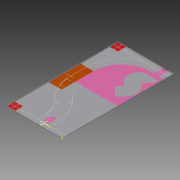
# Autodesk Inventor part: フィールド
Saved by Autodesk Inventor 2015 (Build 190159000, 159)
## iProperties
Created: 2015-08-24
Part Number: フィールド
Material: 一般
Document SubType Name: Modeling
Designer: nobuhiro
Density: 1 g/cm^3
Appearance: 既定
Author: nobuhiro
Autodesk Inventor part; units mm, degrees
ref_plane "YZ Plane" through (0, 0, 0) normal (1, 0, 0) x (0, 1, 0)
ref_plane "XZ Plane" through (0, 0, 0) normal (0, 1, 0) x (-1, 0, 0)
ref_plane "XY Plane" through (0, 0, 0) normal (0, 0, 1) x (1, 0, 0)
sketch "スケッチ1" plane through (0, 0, 0) normal (0, 0, 1) x (1, 0, 0)
  line L0 (7055, 13900) -> (-6950, 13900)
  line L1 (-6950, 13900) -> (-6950, 0)
  line L2 (-7000, -50) -> (0, -50)
  line L3 (0, 13950) -> (-7000, 13950)
  line L4 (-7000, 13950) -> (-7000, -50)
  line L5 (-25, 0) -> (0, 0)
  line L6 (130, 13900) -> (-25, 13900)
  line L7 (-25, 13900) -> (-25, 0)
  line L8 (0, -50) -> (0, 13950)
  line L9 (-6950, 0) -> (0, 0)
  point P0 (52.5, 13900)
  point P1 (52.5, 13900)
  dimension "d4" = 50
  dimension "d17" = 50
  dimension "d18" = 25
  dimension "d176" = 50
  dimension "d177" = 14000
  dimension "d178" = 7000
  constraints: 20 end point, 3 coincident, 3 parallel, 3 point on line, 2 horizontal, 2 midpoint
  measures "d4" distance between parallel lines of L3 L0
  measures "d17" distance between parallel lines of L2 L9
  measures "d18" distance between parallel lines of L8 L7
  measures "d176" distance between parallel lines of L4 L1
  measures "d177" distance of L3.end L2.start
  measures "d178" distance of L2.start L2.end
extrude "押し出し1" add sketch "スケッチ1" against normal blind 1
sketch "スケッチ2" plane through (0, 0, 0) normal (0, 0, 1) x (1, 0, 0)
  line L0 (0, 13950) -> (-7000, 13950) projected
  line L1 (-7000, 13950) -> (-7000, -50) projected
  line L2 (-7000, -50) -> (0, -50) projected
  line L3 (0, 0) -> (-6950, 0)
  line L4 (-6950, 0) -> (-6950, 13900)
  line L5 (-6950, 13900) -> (0, 13900)
  line L6 (-25, -50) -> (-25, 13950)
  line L7 (0, -50) -> (0, 13950) projected
  line L8 (-25, 13950) -> (0, 13950)
  line L9 (0, 13950) -> (0, -50)
  line L10 (0, -50) -> (-25, -50)
  line L11 (0, 0) -> (0, -50)
  line L12 (0, 13900) -> (0, 13950)
  point P0 (0, 0)
  dimension "d7" = 50
  dimension "d8" = 25
  constraints: 18 end point, 3 vertical, 2 point on line, 1 horizontal, 1 parallel, 1 perpendicular, 2 other
  measures "d7" distance between parallel lines of L2 L3
  measures "d8" distance between parallel lines of L7 L6
extrude "押し出し2" add sketch "スケッチ2" along normal blind 50 contours L7 L5 L6 L0 | L6 L5 L4 L3 L2 L1 L0 | L7 L3 L6 L5 | L7 L2 L6 L3
sketch "スケッチ3" plane through (0, 0, 0) normal (0, 0, 1) x (1, 0, 0)
  line L0 (-25, 13900) -> (-6950, 13900) projected
  line L1 (-6950, 0) -> (-25, 0) projected
  line L2 (-25, 0) -> (-25, 13900) projected
  line L3 (-6950, 0) -> (-5950, 0)
  line L4 (-5950, 0) -> (-5950, 1000)
  line L5 (-5950, 1000) -> (-6950, 1000)
  line L6 (-6950, 1000) -> (-6950, 0)
  line L7 (-6950, 0) -> (-6950, 13900) projected
  line L8 (-6950, 5250) -> (-5350, 5250)
  line L9 (-5350, 5250) -> (-5350, 9250)
  line L10 (-5350, 9250) -> (-6950, 9250)
  line L11 (-6950, 9250) -> (-6950, 5250)
  line L12 (-25, 12745) -> (-2037.016, 12745)
  line L13 (-5350, 6950) -> (-25, 6950)
  arc A0 (-2037.016, 12745) -> (-5350, 9250) centre (-1850, 9250) ccw
  line L14 (-700, 12745) -> (-1300, 12745)
  line L15 (-1300, 12745) -> (-1300, 13900)
  line L16 (-1300, 13900) -> (-700, 13900)
  line L17 (-700, 13900) -> (-700, 12745)
  line L18 (-1000, 13900) -> (-1000, 12745)
  line L19 (-6950, 13900) -> (-5950, 13900)
  line L20 (-5950, 13900) -> (-5950, 12900)
  line L21 (-5950, 12900) -> (-6950, 12900)
  line L22 (-6950, 12900) -> (-6950, 13900)
  line L23 (-3131, 1718) -> (-2531, 1718)
  line L24 (-2531, 1718) -> (-2531, 718)
  line L25 (-2531, 718) -> (-3131, 718)
  line L26 (-3131, 718) -> (-3131, 1718)
  line L27 (-2831, 718) -> (-2831, 1718)
  line L28 (-3131, 1718) -> (-2551.4445, 1873.2914)
  line L29 (-2531, 1718) -> (-2551.4445, 1873.2914)
  line L30 (-7000, -50) -> (0, -50) projected
  line L31 (0, 13950) -> (-7000, 13950) projected
  line L32 (0, -50) -> (0, 13950) projected
  point P0 (0, 0)
  dimension "d11" = 1000
  dimension "d12" = 1000
  dimension "d13" = 4000
  dimension "d26" = 300
  dimension "d29" = 1000
  dimension "d30" = 1000
  dimension "d70" = 600
  dimension "d71" = 1000
  dimension "d72" = 4119
  dimension "d73" = 718
  dimension "d74" = 600
  dimension "d75" = 15
  dimension "d170" = 5100
  dimension "d171" = 3500
  dimension "d174" = 50
  dimension "d175" = 4650
  dimension "d179" = 7000
  dimension "d180" = 2300
  dimension "d181" = 1600
  dimension "d182" = 4700
  dimension "d184" = 5650
  dimension "d185" = 1000
  dimension "d191" = 1155
  constraints: 52 end point, 10 parallel, 7 horizontal, 5 midpoint, 5 perpendicular, 5 point on line, 2 point on circle, 1 centre point
  measures "d11" distance of L5.end L4.end
  measures "d12" distance of L4.end L3.end
  measures "d13" distance between parallel lines of L8 L10
  measures "d26" distance between parallel lines of L15 L18
  measures "d29" distance of L20.end L21.end
  measures "d30" distance of L19.end L20.end
  measures "d70" distance of L24.end L25.end
  measures "d71" distance of L25.end L23.start
  measures "d72" distance between parallel lines of L7 L27
  measures "d73" distance between parallel lines of L1 L25
  measures "d74" distance of L23.start L28.end
  measures "d75" angle of L23 L28
  measures "d170" distance from line of L7 A0.centre
  measures "d171" radius of A0
  measures "d174" distance between parallel lines of L31 L0
  measures "d175" distance between parallel lines of L10 L0
  measures "d179" distance between parallel lines of L30 L13
  measures "d180" distance between parallel lines of L10 L13
  measures "d181" distance between parallel lines of L7 L9
  measures "d182" distance between parallel lines of L31 L10
  measures "d184" distance between parallel lines of L7 L15
  measures "d185" distance between parallel lines of L32 L18
  measures "d191" distance between parallel lines of L0 L12
extrude "押し出し3" add sketch "スケッチ3" along normal blind 0.1 contours L17 L12 L18 L0 | L2 L13 L9 A0 L12 | L18 L12 L15 L0 | L9 L8 L7 L10 | L20 L21 L7 L0 | L1 L6 L5 L4 | L28 L29 L23 | L23 L27 L25 L26 | L23 L24 L25 L27
sketch "スケッチ5" plane through (0, 0, 0) normal (0, 0, 1) x (1, 0, 0)
  line L0 (-5350, 5250) -> (-6950, 5250) projected
  line L1 (-6950, 5250) -> (-6950, 1000) projected
  line L2 (-6950, 1000) -> (-5950, 1000) projected
  line L3 (-5950, 1000) -> (-5950, 0) projected
  line L4 (-5950, 0) -> (-25, 0) projected
  line L5 (-25, 0) -> (-25, 6950) projected
  line L6 (-25, 6950) -> (-5350, 6950) projected
  line L7 (-5350, 6950) -> (-5350, 5250) projected
  line L8 (-6950, 9250) -> (-5350, 9250) projected
  arc A0 (-2037.016, 12745) -> (-5350, 9250) centre (-1850, 9250) ccw projected
  line L9 (-2037.016, 12745) -> (-1300, 12745) projected
  line L10 (-1300, 12745) -> (-1300, 13900) projected
  line L11 (-1300, 13900) -> (-5950, 13900) projected
  line L12 (-5950, 13900) -> (-5950, 12900) projected
  line L13 (-5950, 12900) -> (-6950, 12900) projected
  line L14 (-6950, 12900) -> (-6950, 9250) projected
  line L15 (-6950, 13900) -> (-25, 13900) projected
  line L16 (-700, 13900) -> (-700, 12745) projected
  line L17 (-700, 12745) -> (-25, 12745) projected
  line L18 (-25, 12745) -> (-25, 13900) projected
  line L19 (-25, 13900) -> (-700, 13900) projected
  line L20 (-25, 0) -> (-6950, 0) projected
  line L21 (-6950, 0) -> (-6950, 13900) projected
  line L22 (-25, 13900) -> (-25, 0) projected
  line L23 (-6950, 515) -> (-25, 515)
  line L24 (-25, 515) -> (-25, 485)
  line L25 (-25, 485) -> (-6950, 485)
  line L26 (-6950, 485) -> (-6950, 515)
  line L27 (-6465, 0) -> (-6435, 0)
  line L28 (-6435, 0) -> (-6435, 1000)
  line L29 (-6435, 1000) -> (-6465, 1000)
  line L30 (-6465, 1000) -> (-6465, 0)
  line L31 (-2831, 0) -> (-2831, 1718) construction
  line L32 (-2031, 0) -> (-2031, 1718) construction
  line L33 (-3631, 0) -> (-3631, 1584.0254) construction
  line L34 (-2831, 718) -> (-3131, 718) construction
  line L35 (-3131, 718) -> (-3131, 1718) construction
  line L36 (-3631, 1584.0254) -> (-3131, 1718) construction
  line L37 (-2085.5187, 1998.1359) -> (-2031, 1718) construction
  line L38 (-2031, 1718) -> (-3131, 1718) construction
  line L39 (-3131, 1718) -> (-3131, 718) projected
  line L40 (-3131, 718) -> (-2531, 718) projected
  line L41 (-2531, 718) -> (-2531, 1718) projected
  line L42 (-2531, 1718) -> (-2551.4445, 1873.2914) projected
  line L43 (-2551.4445, 1873.2914) -> (-3131, 1718) projected
  line L44 (-3131, 1718) -> (-3415.7009, 2780.5184) construction
  line L45 (-3901.2121, 2650.4261) -> (-2370.2196, 3060.6543) construction
  line L46 (-2836.1455, 2935.8098) -> (-2541.4344, 1835.9332) construction
  line L47 (-3415.7009, 2780.5184) -> (-3965.7009, 3733.1464) construction
  line L48 (-3965.7009, 3733.1464) -> (-4743.5184, 4510.9638) construction
  line L49 (-5109.918, 4144.5642) -> (-4319.2543, 4935.2279) construction
  line L50 (-4319.2543, 4935.2279) -> (-3541.4369, 4157.4104) construction
  line L51 (-3200.3555, 4498.4918) -> (-3965.7009, 3733.1464) construction
  line L52 (-3541.4369, 4157.4104) -> (-3446.0857, 4033.1464) construction
  line L53 (-3446.0857, 4033.1464) -> (-2896.0857, 3080.5184) construction
  line L54 (-2896.0857, 3080.5184) -> (-2836.1455, 2935.8098) construction
  line L55 (-3446.0857, 4033.1464) -> (-3965.7009, 3733.1464) construction
  line L56 (-3415.7009, 2780.5184) -> (-2896.0857, 3080.5184) construction
  line L57 (-4319.2543, 4935.2279) -> (-4869.2543, 5887.8558) construction
  line L58 (-4869.2543, 5887.8558) -> (-5153.9553, 6950.3742) construction
  line L59 (-5153.9553, 6950.3742) -> (-5733.5108, 6795.0828) construction
  line L60 (-5733.5108, 6795.0828) -> (-5448.8098, 5732.5644) construction
  line L61 (-5448.8098, 5732.5644) -> (-4869.2543, 5887.8558) construction
  line L62 (-4743.5184, 4510.9638) -> (-4838.8696, 4635.2279) construction
  line L63 (-4838.8696, 4635.2279) -> (-5388.8696, 5587.8558) construction
  line L64 (-5388.8696, 5587.8558) -> (-5448.8098, 5732.5644) construction
  line L65 (-5388.8696, 5587.8558) -> (-4869.2543, 5887.8558) construction
  line L66 (-4838.8696, 4635.2279) -> (-4319.2543, 4935.2279) construction
  line L67 (-2831, 1718) -> (-2841.2223, 1795.6457) construction
  line L68 (-2841.2223, 1795.6457) -> (-3125.946, 2858.158) construction
  line L69 (-3125.946, 2858.158) -> (-3155.8933, 2930.5184) construction
  line L70 (-3155.8933, 2930.5184) -> (-3705.8933, 3883.1464) construction
  line L71 (-3705.8933, 3883.1464) -> (-3765.5456, 3933.3017) construction
  line L72 (-3765.5456, 3933.3017) -> (-4543.363, 4711.1192) construction
  line L73 (-4543.363, 4711.1192) -> (-4579.062, 4785.2279) construction
  line L74 (-4579.062, 4785.2279) -> (-5129.062, 5737.8558) construction
  line L75 (-5159.0321, 5810.2101) -> (-5129.062, 5737.8558) construction
  line L76 (-5159.0321, 5810.2101) -> (-5443.733, 6872.7285) construction
  line L77 (-2846, -45) -> (-2846, 1717.0168)
  line L78 (-2846, 1717.0168) -> (-2855.8362, 1791.7299)
  line L79 (-2816, -45) -> (-2816, 1718.9832)
  line L80 (-2816, 1718.9832) -> (-2826.6083, 1799.5615)
  line L81 (-2846, -45) -> (-2816, -45)
  line L82 (-2855.8362, 1791.7299) -> (-2826.6083, 1799.5615)
  line L83 (-3631, 1584.0254) -> (-3915.1898, 2644.6363) construction
  line L84 (-3915.1898, 2644.6363) -> (-4332.1005, 3366.7468) construction
  line L85 (-3965.7009, 3733.1464) -> (-4332.1005, 3366.7468) construction
  line L86 (-3131, 1718) -> (-2551.4445, 1873.2914) construction
  line L87 (-2551.4445, 1873.2914) -> (-2085.5187, 1998.1359) construction
  line L88 (-4332.1005, 3366.7468) -> (-5109.918, 4144.5642) construction
  line L89 (-5109.918, 4144.5642) -> (-5949.3209, 5598.4528) construction
  line L90 (-5949.3209, 5598.4528) -> (-5448.8098, 5732.5644) construction
  line L91 (-5949.3209, 5598.4528) -> (-6253.9553, 6735.3637) construction
  line L92 (-5753.9553, 6950.3742) -> (-5753.9553, 7550.3742) construction
  line L93 (-5753.9553, 6950.3742) -> (-5733.5108, 6795.0828) construction
  line L94 (-6253.9553, 6735.3637) -> (-6253.9553, 9250) construction
  line L95 (-5753.9553, 7250.3742) -> (-6950, 7250.3742) construction
  line L96 (-6253.9553, 6950.3742) -> (-5153.9553, 6950.3742) construction
  line L97 (-6950, 13415) -> (-25, 13415)
  line L98 (-25, 13415) -> (-25, 13385)
  line L99 (-25, 13385) -> (-6950, 13385)
  line L100 (-6950, 13385) -> (-6950, 13415)
  line L101 (-6435, 12900) -> (-6465, 12900)
  line L102 (-6465, 12900) -> (-6465, 13900)
  line L103 (-6465, 13900) -> (-6435, 13900)
  line L104 (-6435, 13900) -> (-6435, 12900)
  arc A1 (-3357.8752, 13385) -> (-6253.9553, 9250) centre (-1853.9553, 9250) ccw construction
  line L105 (-1015, 12745) -> (-985, 12745)
  line L106 (-985, 12745) -> (-985, 13900)
  line L107 (-985, 13900) -> (-1015, 13900)
  line L108 (-1015, 13900) -> (-1015, 12745)
  arc A2 (-3401.2109, 13385) -> (-6268.9553, 9250) centre (-1853.9553, 9250) ccw
  line L109 (-6268.9553, 9250) -> (-6268.9553, 6733.3889)
  line L110 (-6268.9553, 6733.3889) -> (-5963.2987, 5592.6631)
  arc A3 (-3313.4072, 13385) -> (-6238.9553, 9250) centre (-1853.9553, 9250) ccw
  line L111 (-6238.9553, 9250) -> (-6238.9553, 6737.3385)
  line L112 (-6238.9553, 6737.3385) -> (-5938.7143, 5616.824)
  line L113 (-5938.7143, 5616.824) -> (-5368.1965, 5769.6938)
  line L114 (-3313.4072, 13385) -> (-3401.2109, 13385)
  line L115 (-5963.2987, 5592.6631) -> (-5121.921, 4135.354)
  line L116 (-5121.921, 4135.354) -> (-4344.1035, 3357.5366)
  line L117 (-5926.5564, 5589.0235) -> (-5097.915, 4153.7745)
  line L118 (-5097.915, 4153.7745) -> (-4332.1005, 3387.96)
  line L119 (-4332.1005, 3387.96) -> (-3974.9251, 3745.1354)
  line L120 (-5926.5564, 5589.0235) -> (-5443.0201, 5718.5866)
  line L121 (-4344.1035, 3357.5366) -> (-3929.1676, 2638.8465)
  line L122 (-3929.1676, 2638.8465) -> (-3646, 1582.0506)
  line L123 (-3937.3264, 3740.3077) -> (-4313.3552, 3364.2789)
  line L124 (-4313.3552, 3364.2789) -> (-3901.2121, 2650.4261)
  line L125 (-3901.2121, 2650.4261) -> (-3620.3934, 1602.3966)
  line L126 (-3620.3934, 1602.3966) -> (-3082.5797, 1746.5033)
  line L127 (-3646, -45) -> (-3646, 1582.0506)
  line L128 (-3616, -45) -> (-3616, 1572.5155)
  line L129 (-3616, 1572.5155) -> (-3131, 1702.4709)
  line L130 (-3620.3934, 1602.3966) -> (-3134.9681, 1732.7466)
  line L131 (-3616, 1572.5155) -> (-3131, 1702.4709)
  line L132 (-3131, 1702.4709) -> (-3131, 1718)
  line L133 (-3937.3264, 3740.3077) -> (-3974.9251, 3745.1354)
  line L134 (-6950, 7265.3742) -> (-5753.9553, 7265.3742)
  line L135 (-5753.9553, 7265.3742) -> (-5753.9553, 7235.3742)
  line L136 (-5753.9553, 7235.3742) -> (-6950, 7235.3742)
  line L137 (-6950, 7235.3742) -> (-6950, 7265.3742)
  line L138 (-3646, -45) -> (-3616, -45)
  line L139 (-2085.5187, 1998.1359) -> (-2370.2196, 3060.6543) construction
  line L140 (-2370.2196, 3060.6543) -> (-3200.3555, 4498.4918) construction
  line L141 (-3200.3555, 4498.4918) -> (-3978.173, 5276.3093) construction
  line L142 (-3978.173, 5276.3093) -> (-4403.3285, 6012.7003) construction
  line L143 (-4403.3285, 6012.7003) -> (-4688.0295, 7075.2187) construction
  line L144 (-4319.2543, 4935.2279) -> (-3978.173, 5276.3093) construction
  line L145 (-4869.2543, 5887.8558) -> (-4403.3285, 6012.7003) construction
  line L146 (-3897.3298, 2635.9372) -> (-3411.8187, 2766.0295)
  line L147 (-3423.4655, 2793.967) -> (-3908.9766, 2663.8747)
  line L148 (-3411.8187, 2766.0295) -> (-3415.7009, 2780.5184)
  line L149 (-3423.4655, 2793.967) -> (-3415.7009, 2780.5184)
  line L150 (-5088.7048, 4144.5642) -> (-4732.9118, 4500.3572)
  line L151 (-4752.7286, 4522.9668) -> (-5106.7018, 4168.9936)
  line L152 (-4732.9118, 4500.3572) -> (-4743.5184, 4510.9638)
  line L153 (-4743.5184, 4510.9638) -> (-4752.7286, 4522.9668)
  line L154 (-2099.7752, 1994.3158) -> (-2046, 1718)
  line L155 (-5950, 0) -> (-25, 0) projected
  line L156 (-2046, 0) -> (-2046, 1718)
  line L157 (-2099.7752, 1994.3158) -> (-2384.4762, 3056.8343)
  line L158 (-3210.792, 4488.0553) -> (-2384.4762, 3056.8343)
  line L159 (-3210.792, 4488.0553) -> (-3988.6095, 5265.8727)
  line L160 (-3988.6095, 5265.8727) -> (-4417.5851, 6008.8802)
  line L161 (-4711.8435, 7107.0675) -> (-4417.5851, 6008.8802)
  line L162 (-2016, 0) -> (-2016, 1720.8921)
  line L163 (-2016, 1720.8921) -> (-2070.5272, 2001.0718)
  line L164 (-2070.5272, 2001.0718) -> (-2356.5206, 3068.4138)
  line L165 (-2356.5206, 3068.4138) -> (-3186.7861, 4506.4757)
  line L166 (-3186.7861, 4506.4757) -> (-3964.6035, 5284.2932)
  line L167 (-3964.6035, 5284.2932) -> (-4389.6295, 6020.4598)
  line L168 (-4389.6295, 6020.4598) -> (-4682.8657, 7114.8321)
  line L169 (-4711.8435, 7107.0675) -> (-4682.8657, 7114.8321)
  line L170 (-2046, 0) -> (-2016, 0)
  line L171 (-2549.4697, 1858.2914) -> (-2096.9028, 1979.5564)
  line L172 (-2103.6575, 2008.8047) -> (-2555.3268, 1887.7803)
  line L173 (-2549.4697, 1858.2914) -> (-2555.3268, 1887.7803)
  line L174 (-2832.2632, 2921.3209) -> (-2380.5939, 3042.3454)
  line L175 (-2392.2408, 3070.2829) -> (-2841.9352, 2949.7876)
  line L176 (-2832.2632, 2921.3209) -> (-2841.9352, 2949.7876)
  line L177 (-3532.2267, 4145.4074) -> (-3203.0275, 4474.6066)
  line L178 (-3221.3986, 4498.6619) -> (-3552.0435, 4168.017)
  line L179 (-3532.2267, 4145.4074) -> (-3552.0435, 4168.017)
  line L180 (-4308.6477, 4924.6213) -> (-3978.0029, 5255.2661)
  line L181 (-3996.3741, 5279.3214) -> (-4327.0189, 4948.6765)
  line L182 (-4327.0189, 4948.6765) -> (-4319.2543, 4935.2279)
  line L183 (-4319.2543, 4935.2279) -> (-4308.6477, 4924.6213)
  line L184 (-4861.4898, 5874.4072) -> (-4409.8205, 5995.4316)
  line L185 (-4421.4674, 6023.3691) -> (-4873.1366, 5902.3447)
  line L186 (-4861.4898, 5874.4072) -> (-4869.2543, 5887.8558)
  line L187 (-4873.1366, 5902.3447) -> (-4869.2543, 5887.8558)
  line L188 (-3131, 1718) -> (-3134.9681, 1732.7466)
  line L189 (-3131, 718) -> (-2531, 718) projected
  line L190 (-5729.6285, 6780.5939) -> (-6215.6507, 6650.3647)
  line L191 (-6223.4153, 6679.3424) -> (-5735.4856, 6810.0828)
  line L192 (-5733.5108, 6795.0828) -> (-6219.533, 6664.8535)
  line L193 (-5443.0201, 5718.5866) -> (-5368.1965, 5769.6938)
  line L194 (-1000, 12745) -> (-1000, 13900)
  line L195 (-5735.4856, 6810.0828) -> (-5729.6285, 6780.5939)
  point P0 (0, 0)
  point P1 (-6465, 500)
  point P2 (-6950, 500)
  point P3 (-6450, 1000)
  point P4 (-6450, 0)
  point P5 (-6435, 13400)
  point P6 (-6950, 13400)
  point P7 (-6450, 12900)
  point P8 (-6450, 12900)
  point P9 (-6224.9553, 5250)
  point P10 (-6238.9553, 6950.3742)
  point P11 (-5330.3035, 5446.4649)
  dimension "d31" = 30
  dimension "d33" = 800
  dimension "d34" = 800
  dimension "d38" = 4119
  dimension "d60" = 1000
  dimension "d68" = 300
  dimension "d69" = 1600
  dimension "d76" = 600
  dimension "d78" = 600
  dimension "d79" = 600
  dimension "d80" = 15
  dimension "d81" = 15
  dimension "d82" = 1100
  dimension "d83" = 1100
  dimension "d84" = 15
  dimension "d85" = 15
  dimension "d86" = 1100
  dimension "d87" = 1100
  dimension "d88" = 15
  dimension "d89" = 15
  dimension "d90" = 30
  dimension "d91" = 15
  dimension "d94" = 15
  dimension "d95" = 15
  dimension "d96" = 600
  dimension "d97" = 600
  dimension "d98" = 500
  dimension "d100" = 30
  dimension "d103" = 15
  dimension "d104" = 15
  dimension "d105" = 15
  dimension "d106" = 15
  dimension "d107" = 15
  dimension "d108" = 15
  dimension "d109" = 15
  dimension "d110" = 15
  dimension "d111" = 15
  dimension "d115" = 30
  dimension "d116" = 15
  dimension "d117" = 4400
  dimension "d118" = 30
  dimension "d119" = 30
  dimension "d120" = 30
  dimension "d122" = 30
  dimension "d123" = 30
  dimension "d124" = 30
  dimension "d125" = 30
  dimension "d126" = 30
  dimension "d127" = 30
  dimension "d166" = 15
  dimension "d167" = 600
  dimension "d168" = 30
  dimension "d169" = 1100
  dimension "d186" = 30
  dimension "d187" = 30
  dimension "d188" = 1155
  dimension "d189" = 300
  dimension "d190" = 30
  constraints: 335 end point, 76 point on line, 43 parallel, 19 perpendicular, 18 midpoint, 11 collinear, 11 horizontal, 9 equal length, 6 point on circle, 4 vertical, 3 centre point, 2 horizontal alignment, 1 coincident, 1 tangent, 1 vertical alignment, 28 other
  measures "d31" distance between parallel lines of L25 L23
  measures "d33" distance between parallel lines of L31 L33
  measures "d34" distance between parallel lines of L31 L32
  measures "d38" distance between parallel lines of L1 L31
  measures "d60" distance of L34.end L35.end
  measures "d68" distance between parallel lines of L31 L35
  measures "d69" distance of L33.end L37.start
  measures "d76" distance between parallel lines of L44 L46
  measures "d78" distance between parallel lines of L53 L47
  measures "d79" distance between parallel lines of L50 L48
  measures "d80" angle of L45 L56
  measures "d81" angle of L55 L51
  measures "d82" distance of L52.end L53.end
  measures "d83" distance between parallel lines of L51 L49
  measures "d84" angle of L66 L49
  measures "d85" angle of L65 L61
  measures "d86" distance of L49.end L57.end
  measures "d87" distance of L57.end L58.end
  measures "d88" distance between parallel lines of L31 L77
  measures "d89" distance between parallel lines of L31 L79
  measures "d90" distance between parallel lines of L80 L78
  measures "d91" distance between parallel lines of L78 L67
  measures "d94" angle of L87 L38
  measures "d95" angle of L38 L36
  measures "d96" distance of L92.start L92.end
  measures "d97" distance from line of L92 L58.end
  measures "d98" distance between parallel lines of L92 L94
  measures "d100" distance between parallel lines of L97 L99
  measures "d103" distance between parallel lines of L91 L110
  measures "d104" distance between parallel lines of L91 L112
  measures "d105" distance between parallel lines of L89 L115
  measures "d106" distance between parallel lines of L89 L117
  measures "d107" distance between parallel lines of L84 L121
  measures "d108" distance between parallel lines of L84 L124
  measures "d109" distance between parallel lines of L88 L116
  measures "d110" distance between parallel lines of L33 L127
  measures "d111" distance between parallel lines of L33 L128
  measures "d115" radial gap between concentric circles of A2 A3
  measures "d116" radial gap between concentric circles of A2 A1
  measures "d117" radius of A1
  measures "d118" distance between parallel lines of L125 L122
  measures "d119" distance between parallel lines of L147 L146
  measures "d120" distance between parallel lines of L151 L150
  measures "d122" distance between parallel lines of L156 L162
  measures "d123" distance between parallel lines of L172 L171
  measures "d124" distance between parallel lines of L175 L174
  measures "d125" distance between parallel lines of L178 L177
  measures "d126" distance between parallel lines of L180 L181
  measures "d127" distance between parallel lines of L185 L184
  measures "d166" angle of L96 L59
  measures "d167" distance between parallel lines of L58 L60
  measures "d168" distance between parallel lines of L191 L190
  measures "d169" distance of L39.start L44.end
  measures "d186" distance between parallel lines of L113 L120
  measures "d187" distance between parallel lines of L109 L111
  measures "d188" distance between parallel lines of L15 L105
  measures "d189" distance between parallel lines of L16 L194
  measures "d190" distance between parallel lines of L108 L106
extrude "押し出し4" add sketch "スケッチ5" along normal blind 0.2 contours L117 L118 L119 L133 L123 L124 L125 L126 L188 L39 L129 L128 L23 L127 L122 L121 L116 L115 L0 | L0 L115 L110 L109 L136 L111 L112 L113 L193 L120 L117 | L151 L153 L152 L150 L118 L117 | L161 L169 L168 L6 | L6 L168 L167 L166 L165 L164 L163 L162 L23 L156 L154 L157 L158 L159 L160 L161 | L161 L160 L184 L186 L187 L185 | L21 L134 L109 L136 | L2 L28 L23 L30 | L23 L30 L25 L21 | L109 L134 L111 L136 | L5 L25 L162 L23 | L23 L28 L25 L30 | L109 L8 L111 L134 | L111 L134 L135 L136 | L112 L191 L195 L190 | L162 L25 L156 L23 | L99 L16 L97 L18 | L160 L159 L180 L183 L182 L181 | L23 L3 L25 L28 | L25 L28 L20 L30 | A2 L99 A3 L8 | L127 L25 L3 L23 | L23 L128 L25 L127 | L162 L4 L156 L25 | L156 L25 L79 L23 | L99 L106 L97 L16 | L99 L12 L97 L10 | L102 L99 L104 L13 | L21 L97 L102 L99 | L23 L77 L25 L128 | L25 L128 L4 L127 | L79 L25 L77 L23 | L23 L77 L40 L79 | L106 L105 L194 L99 | L99 L194 L97 L106 | L99 L104 L97 L12 | L102 L97 L104 L99 | L4 L128 L138 L127 | L147 L149 L148 L146 L125 L124 | L79 L4 L77 L25 | L40 L77 L78 L43 L80 L79 | L171 L42 L43 L173 L172 L157 L154 | L97 L194 L15 L106 | L194 L105 L108 L99 | L99 L108 L97 L194 | L159 L158 L177 L179 L178 | L10 L97 L108 L99 | L102 L15 L104 L97 | L79 L81 L77 L4 | L173 L43 L42 | L97 L108 L15 L194 | L126 L130 L188 | L174 L176 L175 L158 L157
sketch "スケッチ6" plane through (0, 0, 0.1) normal (0, 0, 1) x (1, 0, 0)
  line L0 (-25, 12745) -> (-700, 12745) projected
  line L1 (-1594.8055, 10819.0057) -> (-966.5332, 10176.2685) projected
  arc A0 (-974.2542, 8819.3618) -> (-966.5332, 10176.2685) centre (-1656.6122, 9501.7198) ccw projected
  line L2 (-974.2542, 8819.3618) -> (-1171.8961, 8621.7198) projected
  line L3 (-2020.4243, 8621.7198) -> (-1396.7505, 9245.3936) projected
  arc A1 (-1396.7505, 9245.3936) -> (-1393.3525, 9754.6024) centre (-1653.0767, 9501.7198) ccw projected
  line L4 (-1393.3525, 9754.6024) -> (-2023.3007, 10401.5935) projected
  arc A2 (-1951.2153, 11706.1364) -> (-2023.3007, 10401.5935) centre (-1387.4243, 11020.7198) ccw projected
  line L5 (-1951.2153, 11706.1364) -> (-1504.3852, 12073.6776) projected
  arc A3 (-1504.3852, 12073.6776) -> (-1307.4243, 12490.7198) centre (-1847.4243, 12490.7198) ccw projected
  line L6 (-1307.4243, 12490.7198) -> (-1307.4243, 12790.7198) projected
  line L7 (-707.4243, 12790.7198) -> (-707.4243, 12490.7198) projected
  arc A4 (-1153.1063, 11574.3102) -> (-707.4243, 12490.7198) centre (-1872.4243, 12490.7198) ccw projected
  line L8 (-1153.1063, 11574.3102) -> (-1566.482, 11249.839) projected
  arc A5 (-1566.482, 11249.839) -> (-1594.8055, 10819.0057) centre (-1387.4243, 11021.7198) ccw projected
  line L9 (-2373.9777, 8975.2732) -> (-1242.6068, 7843.9024)
  line L10 (-2373.9777, 8975.2732) -> (-1846.242, 9503.0088)
  line L11 (-1846.242, 9503.0088) -> (-2381.541, 10052.7899)
  arc A6 (-2268.8441, 12092.2866) -> (-2381.541, 10052.7899) centre (-1387.4243, 11020.7198) ccw
  line L12 (-2268.8441, 12092.2866) -> (-2083.1861, 12245)
  arc A7 (-844.3861, 11181.0013) -> (-225.6557, 12245) centre (-1872.4243, 12490.7198) ccw
  line L13 (-844.3861, 11181.0013) -> (-1073.595, 11001.0883)
  line L14 (-1073.595, 11001.0883) -> (-608.9793, 10525.7757)
  arc A8 (-620.7008, 8465.8084) -> (-608.9793, 10525.7757) centre (-1656.6122, 9501.7198) ccw
  line L15 (-620.7008, 8465.8084) -> (-1242.6068, 7843.9024)
  line L16 (-2083.1861, 12245) -> (-225.6557, 12245)
  point P0 (0, 0)
  dimension "d128" = 500
  dimension "d129" = 500
  dimension "d130" = 500
  dimension "d131" = 500
  dimension "d132" = 500
  constraints: 16 end point, 6 point on circle, 3 centre point, 1 horizontal, 1 perpendicular, 1 point on line, 4 other
  measures "d128" radial gap between concentric circles of A2 A6
  measures "d129" radial gap between concentric circles of A0 A8
  measures "d130" distance between parallel lines of L0 L16
  measures "d131" radial gap between concentric circles of A4 A7
  measures "d132" distance between parallel lines of L12 L5
extrude "押し出し5" add sketch "スケッチ6" along normal blind 0.1
sketch "スケッチ8" plane through (0, 0, 0.1) normal (0, 0, 1) x (1, 0, 0)
  line L0 (-2373.9777, 8975.2732) -> (-1846.242, 9503.0088) projected
  line L1 (-1846.242, 9503.0088) -> (-2381.541, 10052.7899) projected
  arc A0 (-2268.8441, 12092.2866) -> (-2381.541, 10052.7899) centre (-1387.4243, 11020.7198) ccw projected
  line L2 (-2268.8441, 12092.2866) -> (-2083.1861, 12245) projected
  line L3 (-2083.1861, 12245) -> (-225.6557, 12245) projected
  arc A1 (-844.3861, 11181.0013) -> (-225.6557, 12245) centre (-1872.4243, 12490.7198) ccw projected
  line L4 (-844.3861, 11181.0013) -> (-1073.595, 11001.0883) projected
  line L5 (-1073.595, 11001.0883) -> (-608.9793, 10525.7757) projected
  arc A2 (-620.7008, 8465.8084) -> (-608.9793, 10525.7757) centre (-1656.6122, 9501.7198) ccw projected
  line L6 (-620.7008, 8465.8084) -> (-1242.6068, 7843.9024) projected
  line L7 (-1242.6068, 7843.9024) -> (-2373.9777, 8975.2732) projected
  line L8 (-700, 12745) -> (-700, 13385) projected
  line L9 (-1300, 13385) -> (-1300, 12745) projected
  line L10 (-1300, 12745) -> (-2037.016, 12745) projected
  arc A3 (-2037.016, 12745) -> (-5350, 9250) centre (-1850, 9250) ccw projected
  line L11 (-6268.9553, 9250) -> (-6950, 9250) projected
  line L12 (-5730.8211, 5250) -> (-5350, 5250) projected
  line L13 (-5350, 5250) -> (-5350, 6950) projected
  line L14 (-5350, 6950) -> (-4669.7574, 6950) projected
  line L15 (-25, 12745) -> (-25, 6950) projected
  line L16 (-25, 12745) -> (-700, 12745) projected
  line L17 (-5350, 6950) -> (-5350, 9250)
  line L18 (-6950, 7265.3742) -> (-6950, 9250) projected
  line L19 (-5950, 0) -> (-6435, 0) projected
  line L20 (-5950, 0) -> (-5950, 485) projected
  line L21 (-5950, 1000) -> (-6435, 1000) projected
  line L22 (-6950, 0) -> (-6950, 485) projected
  line L23 (-1300, 13900) -> (-1015, 13900) projected
  line L24 (-6950, 5250) -> (-6950, 7235.3742) projected
  line L25 (-6950, 12900) -> (-6465, 12900) projected
  line L26 (-5950, 12900) -> (-5950, 13385) projected
  line L27 (-6950, 13900) -> (-6465, 13900) projected
  line L28 (-985, 13415) -> (-700, 13415) projected
  line L29 (-700, 13415) -> (-700, 13900) projected
  line L30 (-985, 13900) -> (-700, 13900) projected
  line L31 (-985, 13900) -> (-985, 13415) projected
  line L32 (-6465, 485) -> (-6950, 485) projected
  line L33 (-6465, 0) -> (-6950, 0) projected
  line L34 (-6465, 0) -> (-6465, 485) projected
  line L35 (-700, 13385) -> (-985, 13385) projected
  line L36 (-985, 13385) -> (-985, 12745) projected
  line L37 (-985, 12745) -> (-1015, 12745) projected
  line L38 (-1015, 12745) -> (-1015, 13385) projected
  line L39 (-1015, 13385) -> (-1300, 13385) projected
  line L40 (-6238.9553, 9250) -> (-6238.9553, 7265.3742) projected
  line L41 (-6238.9553, 7265.3742) -> (-5753.9553, 7265.3742) projected
  line L42 (-5753.9553, 7265.3742) -> (-5753.9553, 7235.3742) projected
  line L43 (-5753.9553, 7235.3742) -> (-6238.9553, 7235.3742) projected
  line L44 (-6238.9553, 7235.3742) -> (-6238.9553, 6737.3385) projected
  line L45 (-6215.6507, 6650.3647) -> (-5938.7143, 5616.824) projected
  line L46 (-5938.7143, 5616.824) -> (-5368.1965, 5769.6938) projected
  line L47 (-5368.1965, 5769.6938) -> (-5443.0201, 5718.5866) projected
  line L48 (-5443.0201, 5718.5866) -> (-5926.5564, 5589.0235) projected
  line L49 (-5926.5564, 5589.0235) -> (-5730.8211, 5250) projected
  line L50 (-4669.7574, 6950) -> (-4711.8435, 7107.0675) projected
  line L51 (-4711.8435, 7107.0675) -> (-4682.8657, 7114.8321) projected
  line L52 (-4682.8657, 7114.8321) -> (-4638.6991, 6950) projected
  line L53 (-4638.6991, 6950) -> (-25, 6950) projected
  line L54 (-1015, 13415) -> (-1015, 13900) projected
  line L55 (-1300, 13900) -> (-1300, 13415) projected
  line L56 (-1300, 13415) -> (-1015, 13415) projected
  line L57 (-6268.9553, 7265.3742) -> (-6268.9553, 9250) projected
  line L58 (-6950, 7265.3742) -> (-6268.9553, 7265.3742) projected
  line L59 (-6268.9553, 7235.3742) -> (-6950, 7235.3742) projected
  line L60 (-6950, 5250) -> (-5765.4621, 5250) projected
  line L61 (-5765.4621, 5250) -> (-5963.2987, 5592.6631) projected
  line L62 (-5963.2987, 5592.6631) -> (-6268.9553, 6733.3889) projected
  line L63 (-6268.9553, 6733.3889) -> (-6268.9553, 7235.3742) projected
  line L64 (-6435, 485) -> (-6435, 0) projected
  line L65 (-5950, 485) -> (-6435, 485) projected
  line L66 (-6950, 515) -> (-6465, 515) projected
  line L67 (-6465, 515) -> (-6465, 1000) projected
  line L68 (-6465, 1000) -> (-6950, 1000) projected
  line L69 (-6950, 515) -> (-6950, 1000) projected
  line L70 (-6435, 1000) -> (-6435, 515) projected
  line L71 (-6435, 515) -> (-5950, 515) projected
  line L72 (-5950, 515) -> (-5950, 1000) projected
  line L73 (-6950, 13415) -> (-6465, 13415) projected
  line L74 (-6465, 13415) -> (-6465, 13900) projected
  line L75 (-6950, 13415) -> (-6950, 13900) projected
  line L76 (-6465, 13385) -> (-6950, 13385) projected
  line L77 (-6950, 12900) -> (-6950, 13385) projected
  line L78 (-6465, 12900) -> (-6465, 13385) projected
  line L79 (-6435, 13385) -> (-6435, 12900) projected
  line L80 (-6435, 12900) -> (-5950, 12900) projected
  line L81 (-5950, 13385) -> (-6435, 13385) projected
  line L82 (-6435, 13900) -> (-6435, 13415) projected
  line L83 (-6435, 13415) -> (-5950, 13415) projected
  line L84 (-5950, 13415) -> (-5950, 13900) projected
  line L85 (-6435, 13900) -> (-5950, 13900) projected
  line L86 (-6223.4153, 6679.3424) -> (-5735.4856, 6810.0828) projected
  line L87 (-5735.4856, 6810.0828) -> (-5729.6285, 6780.5939) projected
  line L88 (-5729.6285, 6780.5939) -> (-6215.6507, 6650.3647) projected
  line L89 (-6238.9553, 6737.3385) -> (-6223.4153, 6679.3424) projected
  line L90 (-1300, 12745) -> (-700, 12745)
  line L91 (-5350, 9250) -> (-6238.9553, 9250) projected
  point P0 (0, 0)
  constraints: 4 end point, 1 horizontal, 1 vertical
extrude "押し出し7" cut sketch "スケッチ8" against normal blind 0.1 contours L16 L15 L53 L52 L51 L50 L14 L17 A3 L10 L90 L37
sketch "スケッチ7" plane through (0, 0, 0) normal (0, 0, 1) x (1, 0, 0)
  line L0 (-2.5, 14000) -> (-6950, 14000)
  line L1 (-6950, 0) -> (-2.5, 0)
  line L2 (-2.5, 0) -> (-2.5, 14000)
  line L3 (-6950, 0) -> (-5950, 0)
  line L4 (-5950, 0) -> (-5950, 1000)
  line L5 (-5950, 1000) -> (-6950, 1000)
  line L6 (-6950, 1000) -> (-6950, 0)
  line L7 (-6950, 0) -> (-6950, 14000)
  line L8 (-6950, 5250) -> (-5350, 5250)
  line L9 (-5350, 5250) -> (-5350, 9250)
  line L10 (-5350, 9250) -> (-6950, 9250)
  line L11 (-6950, 9250) -> (-6950, 5250)
  line L12 (-2.5, 12745) -> (-1850.0036, 12745)
  line L13 (-5350, 6950) -> (-2.5, 6950)
  arc A0 (-1850.0036, 12745) -> (-5350, 9250) centre (-1850.0036, 9245) ccw
  line L14 (-702.5, 12745) -> (-1302.5, 12745)
  line L15 (-1302.5, 12745) -> (-1302.5, 14000)
  line L16 (-1302.5, 14000) -> (-702.5, 14000)
  line L17 (-702.5, 14000) -> (-702.5, 12745)
  line L18 (-1002.5, 14000) -> (-1002.5, 12745)
  line L19 (-6950, 14000) -> (-5950, 14000)
  line L20 (-5950, 14000) -> (-5950, 13000)
  line L21 (-5950, 13000) -> (-6950, 13000)
  line L22 (-6950, 13000) -> (-6950, 14000)
  line L23 (-3087, 1763) -> (-2487, 1763)
  line L24 (-2487, 1763) -> (-2487, 763)
  line L25 (-2487, 763) -> (-3087, 763)
  line L26 (-3087, 763) -> (-3087, 1763)
  line L27 (-2787, 763) -> (-2787, 1763)
  line L28 (-3087, 1763) -> (-2507.4445, 1918.2914)
  line L29 (-2487, 1763) -> (-2507.4445, 1918.2914)
  line L30 (-6950, 13900) -> (-25, 13900) projected
  line L31 (-7000, -50) -> (0, -50) projected
  line L32 (-6950, 5250) -> (-6950, 1000) projected
  point P0 (0, 0)
  point P1 (0, 0)
  dimension "d135" = 1000
  dimension "d136" = 1000
  dimension "d137" = 4000
  dimension "d138" = 1600
  dimension "d141" = 2300
  dimension "d142" = 3500
  dimension "d143" = 1000
  dimension "d144" = 300
  dimension "d145" = 1000
  dimension "d146" = 1000
  dimension "d147" = 600
  dimension "d148" = 1000
  dimension "d149" = 4163
  dimension "d150" = 763
  dimension "d151" = 600
  dimension "d152" = 15
  dimension "d192" = 1155
  dimension "d193" = 7000
  constraints: 60 end point, 10 parallel, 7 horizontal, 6 point on line, 5 perpendicular, 4 midpoint, 2 point on circle, 1 centre point, 1 collinear, 1 tangent
  measures "d135" distance of L5.end L4.end
  measures "d136" distance of L4.end L3.end
  measures "d137" distance between parallel lines of L8 L10
  measures "d138" distance of L9.end L10.end
  measures "d141" distance between parallel lines of L10 L13
  measures "d142" radius of A0
  measures "d143" distance between parallel lines of L2 L18
  measures "d144" distance between parallel lines of L15 L18
  measures "d145" distance of L20.end L21.end
  measures "d146" distance of L19.end L20.end
  measures "d147" distance of L24.end L25.end
  measures "d148" distance of L25.end L23.start
  measures "d149" distance between parallel lines of L7 L27
  measures "d150" distance between parallel lines of L1 L25
  measures "d151" distance of L23.start L28.end
  measures "d152" angle of L23 L28
  measures "d192" distance between parallel lines of L30 L12
  measures "d193" distance between parallel lines of L31 L13
extrude "押し出し6" add sketch "スケッチ7" along normal blind 0.1 separate body contours L2 L13 L9 A0 L12
sketch "スケッチ9" plane through (0, 0, 0.2) normal (0, 0, 1) x (1, 0, 0)
  circle A0 centre (-1000, 13320) radius 4
  circle A1 centre (-1000, 13270) radius 4
  line L0 (-985, 13415) -> (-1015, 13415)
  line L1 (-1015, 13415) -> (-1015, 13385)
  line L2 (-1015, 13385) -> (-985, 13385)
  line L3 (-985, 13385) -> (-985, 13415)
  line L4 (-985, 13415) -> (-1015, 13385) construction
  line L5 (-1015, 13415) -> (-985, 13385) construction
  circle A2 centre (-920, 13400) radius 4
  circle A3 centre (-870, 13400) radius 4
  circle A4 centre (-1000, 13480) radius 4
  circle A5 centre (-1000, 13530) radius 4
  circle A6 centre (-1080, 13400) radius 4
  circle A7 centre (-1130, 13400) radius 4
  point P0 (0, 0)
  point P1 (-1000, 13400)
  point P2 (-1000, 13400)
  dimension "d157" = 80
  dimension "d158" = 130
  dimension "d159" = 8
  dimension "d162" = 360
  constraints: 12 end point, 8 centre point, 3 midpoint, 2 parallel, 2 vertical alignment, 1 equal radius, 1 horizontal, 1 perpendicular, 17 other
  measures "d157" distance of A0.centre point (-1000, 13400)
  measures "d158" distance of A1.centre point (-1000, 13400)
  measures "d159" diameter of A0
extrude "押し出し8" cut sketch "スケッチ9" against normal through all contours A0 | A1 | A2 | A3 | A4 | A5 | A6 | A7 bodies 1
sketch "スケッチ10" plane through (0, 0, 0.2) normal (0, 0, 1) x (1, 0, 0)
  line L0 (-2816, 0) -> (-2816, 485) projected
  line L1 (-2816, 485) -> (-2046, 485) projected
  line L2 (-1015, 13900) -> (-985, 13900) projected
  point P0 (0, 0)
  point P1 (-2831, 500)
  point P2 (-1000, 13900)
  dimension "d194" = 15
  dimension "d195" = 15
  constraints: 1 midpoint
  measures "d194" distance from line of L0 point (-2831, 500)
  measures "d195" distance from line of point (-2831, 500) L1
equation "\"d78\" = d76"
equation "\"d79\" = d78"
